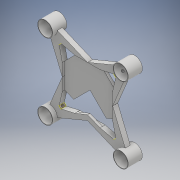
# Autodesk Inventor part: DRONE
Saved by Autodesk Inventor 2018 (Build 220112000, 112)
## iProperties
Created: 2022-03-15
Part Number: DRONE
Material: Genérico
Document SubType Name: Modeling
Designer: ADM
Density: 1 g/cm^3
Appearance: Padrão
Author: ADM
Autodesk Inventor part; units mm, degrees
ref_plane "YZ Plane" through (0, 0, 0) normal (1, 0, 0) x (0, 1, 0)
ref_plane "XZ Plane" through (0, 0, 0) normal (0, 1, 0) x (-1, 0, 0)
ref_plane "XY Plane" through (0, 0, 0) normal (0, 0, 1) x (1, 0, 0)
sketch "Esboço1" plane through (0, 0, 0) normal (0, 1, 0) x (-1, 0, 0)
  line L0 (0, 0) -> (0, -150)
  line L1 (0, 0) -> (150, 0)
  line L2 (150, 0) -> (150, -150)
  line L3 (150, -150) -> (0, -150)
  circle A0 centre (150, -150) radius 15
  circle A1 centre (0, -150) radius 15
  circle A2 centre (0, 0) radius 15
  circle A3 centre (150, 0) radius 15
  line L4 (0, 0) -> (150, -150)
  line L5 (150, 0) -> (0, -150)
  line L6 (75, -75) -> (75, -125)
  line L7 (75, -125) -> (75, -25)
  line L8 (75, -75) -> (125, -75)
  line L9 (75, -25) -> (25, -25)
  line L10 (25, -25) -> (25, -75)
  line L11 (25, -75) -> (25, -125)
  line L12 (25, -125) -> (75, -125)
  line L13 (75, -125) -> (125, -125)
  line L14 (125, -125) -> (125, -75)
  line L15 (125, -75) -> (125, -25)
  line L16 (125, -25) -> (75, -25)
  line L17 (135, -150) -> (75, -125)
  line L18 (125, -75) -> (150, -135)
  line L19 (135, 0) -> (75, -25)
  line L20 (150, -15) -> (125, -75)
  line L21 (15, 0) -> (75, -25)
  line L22 (0, -15) -> (25, -75)
  line L23 (0, -135) -> (25, -75)
  line L24 (15, -150) -> (75, -125)
  line L25 (10.6066, -10.6066) -> (17.6777, -17.6777)
  line L26 (17.6777, -17.6777) -> (50, -25)
  line L27 (17.6777, -17.6777) -> (25, -50)
  line L28 (10.6066, -139.3934) -> (17.6777, -132.3223)
  line L29 (17.6777, -132.3223) -> (25, -100)
  line L30 (17.6777, -132.3223) -> (50, -125)
  line L31 (139.3934, -10.6066) -> (132.3223, -17.6777)
  line L32 (132.3223, -17.6777) -> (100, -25)
  line L33 (132.3223, -17.6777) -> (125, -50)
  line L34 (139.3934, -139.3934) -> (132.3223, -132.3223)
  line L35 (132.3223, -132.3223) -> (125, -100)
  line L36 (132.3223, -132.3223) -> (100, -125)
  dimension "d45" = 150
  dimension "d46" = 150
  dimension "d47" = 150
  dimension "d48" = 30
  dimension "d49" = 30
  dimension "d50" = 30
  dimension "d51" = 30
  dimension "d52" = 50
  dimension "d53" = 100
  dimension "d54" = 50
  dimension "d55" = 100
  dimension "d56" = 50
  dimension "d57" = 50
  dimension "d58" = 50
  dimension "d59" = 50
  dimension "d60" = 10
  dimension "d61" = 10
  dimension "d62" = 10
  dimension "d63" = 10
  constraints: 72 end point, 16 point on line, 12 point on circle, 8 midpoint, 4 centre point, 4 coincident, 2 horizontal, 2 vertical, 1 perpendicular, 10 other
  measures "d45" distance of L0.start L0.end
  measures "d46" distance of L0.start L1.end
  measures "d47" distance of L1.end L2.end
  measures "d48" diameter of A0
  measures "d49" diameter of A1
  measures "d50" diameter of A2
  measures "d51" diameter of A3
  measures "d52" distance of L6.start L6.end
  measures "d53" distance of L6.end L7.end
  measures "d54" distance of L6.start L8.end
  measures "d55" distance of L8.end L10.end
  measures "d56" distance of L7.end L9.end
  measures "d57" distance of L10.end L11.end
  measures "d58" distance of L6.end L13.end
  measures "d59" distance of L8.end L15.end
  measures "d60" distance of L25.start L25.end
  measures "d61" distance of L28.start L28.end
  measures "d62" distance of L31.start L31.end
  measures "d63" distance of L34.start L34.end
extrude "Extrusão1" add sketch "Esboço1" along normal mid plane 28 contours L4 A2 L0 | L0 A2 L1 | L1 A2 L4 | A1 L5 L0 | L0 L3 A1 | A3 L2 L1 | L1 L5 A3 | L5 A1 L3 | L2 A3 L5 | A0 L4 L3 | L3 L2 A0 | L4 A0 L2
extrude "Extrusão2" add sketch "Esboço1" along normal mid plane 10 contours A2 L4 L27 L10 L22 | L21 L9 L26 L4 A2 | L23 L11 L29 L5 A1 | A3 L5 L32 L16 L19 | L5 L30 L12 L24 A1 | A3 L20 L15 L33 L5 | L17 L13 L36 L4 A0 | L18 A0 L4 L35 L14
sketch "Esboço2" plane through (0, -5, 0) normal (0, -1, 0) x (1, 0, 0)
  line L0 (-75, -25) -> (-100, -25) projected
  line L1 (-25.0044, -125) -> (-124.5405, -125)
  line L2 (-132.3223, -132.3223) -> (-125, -100) projected
  line L3 (-17.6777, -132.3223) -> (-25, -100) projected
  line L4 (-125, -50) -> (-125, -75) projected
  line L5 (-125, -50) -> (-74.7992, -75.1004)
  line L6 (-50, -125) -> (-17.6777, -132.3223) projected
  line L7 (-74.7992, -75.1004) -> (-25, -100)
  line L8 (-124.5405, -125) -> (-25.0044, -125)
  line L9 (-74.7725, -125) -> (-25.0044, -125)
  point P0 (0, 0)
  point P1 (-100, -125)
  constraints: 10 end point, 3 collinear, 1 midpoint, 1 parallel
extrude "Extrusão3" add sketch "Esboço1" along normal blind 5 contours L10 L4 L5 L11 | L16 L5 L7 | L7 L4 L9 | L8 L14 L4
extrude "Extrusão4" add sketch "Esboço1" along normal blind 5 contours A3 L20 L15 L33 L5 | L5 L15 L8
sketch "Esboço3" plane through (0, -5, 0) normal (0, -1, 0) x (1, 0, 0)
  line L0 (-100, -125) -> (-75, -125) projected
  line L1 (-75, -125) -> (-75, -115)
  line L2 (-132.3223, -132.3223) -> (-100, -125) projected
  line L3 (-75, -115) -> (-100, -125)
  line L4 (-50, -125) -> (-17.6777, -132.3223) projected
  line L5 (-75, -115) -> (-50, -125)
  point P0 (0, 0)
  dimension "d72" = 10
  constraints: 6 end point, 1 vertical
  measures "d72" distance of L0.end L1.end
extrude "Extrusão5" add sketch "Esboço3" against normal blind 5
sketch "Esboço4" plane through (0, -5, 0) normal (0, -1, 0) x (1, 0, 0)
  line L0 (-75, -125) -> (-75, -115) projected
  line L1 (-50, -125) -> (-17.6777, -132.3223) projected
  line L2 (-75, -115) -> (-50, -125)
  line L3 (-50, -125) -> (-17.6777, -132.3223)
  line L4 (-25, -75) -> (-25, -100) projected
  line L5 (-17.6777, -132.3223) -> (-25, -100)
  line L6 (-25, -125) -> (-124.7945, -125)
  line L7 (-75, -115) -> (-100, -125) projected
  line L8 (-135, -150) -> (-75, -125) projected
  line L9 (-75, -115) -> (-75, -125)
  line L10 (-75, -125) -> (-50, -125)
  line L11 (-75, -125) -> (-50, -125) projected
  line L12 (-50, -125) -> (-75, -125)
  point P0 (0, 0)
  constraints: 14 end point, 1 collinear, 1 horizontal, 1 perpendicular, 1 vertical
extrude "Extrusão6" add sketch "Esboço4" against normal blind 5 contours L0 L2 L6
sketch "Esboço5" plane through (-150, -14, -150) normal (0, -1, 0) x (1, 0, 0)
  circle A0 centre (150, 150) radius 14
  circle A1 centre (-0.0474, 150) radius 14
  circle A2 centre (0, 0) radius 14
  circle A3 centre (150, 0) radius 14
  dimension "d77" = 28
  dimension "d78" = 28
  dimension "d79" = 28
  dimension "d80" = 28
  constraints: 4 centre point, 1 coincident
  measures "d77" diameter of A0
  measures "d78" diameter of A1
  measures "d79" diameter of A2
  measures "d80" diameter of A3
hole "Furo1" at (0, -14, 0) at (-150.0474, -14, 0) at (-150, -14, -150) at (0, -14, -150) direction (0, 1, 0) diameter 28 depth 26 tip angle 118
chamfer "Chanfro1" distance 5 angle 45 4 edges at (-17.6777, 0, -17.6777) (-17.6777, 0, -132.3223) (-132.3223, 0, -132.3223) (-132.3223, 0, -17.6777)
ref_plane "Plano de trabalho1" through (-131.2176, -5, -22.5541) normal (0.7071068, 0, -0.7071068) x (-0.7071068, 0, -0.7071068)
sketch "Esboço6" plane through (-131.2176, -5, -22.5541) normal (0.7071068, 0, -0.7071068) x (-0.7071068, 0, -0.7071068)
  circle A0 centre (-2.6721, 5) radius 2.5
  point P0 (-108.733, 5)
  dimension "d92" = 5
  constraints: 1 centre point
  measures "d92" diameter of A0
hole "Furo2" at (-129.3282, 0, -20.6646) direction (-0.7071068, 0, 0.7071068) diameter 5 depth 20 tip angle 118
ref_plane "Plano de trabalho2" through (-18.7824, -5, -127.4459) normal (-0.7071068, 0, 0.7071068) x (0.7071068, 0, 0.7071068)
sketch "Esboço7" plane through (-18.7824, -5, -127.4459) normal (-0.7071068, 0, 0.7071068) x (0.7071068, 0, 0.7071068)
  circle A0 centre (-2.678, 5) radius 2.5
  point P0 (103.399, 5)
  dimension "d101" = 5
  constraints: 1 centre point
  measures "d101" diameter of A0
hole "Furo3" at (-20.676, 0, -129.3395) direction (0.7071068, 0, -0.7071068) diameter 5 depth 20 tip angle 118
ref_plane "Plano de trabalho3" through (-18.7824, -5, -22.5541) normal (-0.7071068, 0, -0.7071068) x (-0.7071068, 0, 0.7071068)
sketch "Esboço8" plane through (-18.7824, -5, -22.5541) normal (-0.7071068, 0, -0.7071068) x (-0.7071068, 0, 0.7071068)
  circle A0 centre (2.667, 5) radius 2.5
  dimension "d110" = 5
  constraints: 1 centre point, 1 coincident
  measures "d110" diameter of A0
hole "Furo4" at (-20.6682, 0, -20.6682) direction (0.7071068, 0, 0.7071068) diameter 5 depth 20 tip angle 118
ref_plane "Plano de trabalho4" through (-127.4459, -5, -131.2176) normal (0.7071068, 0, 0.7071068) x (0.7071068, 0, -0.7071068)
sketch "Esboço9" plane through (-127.4459, -5, -131.2176) normal (0.7071068, 0, 0.7071068) x (0.7071068, 0, -0.7071068)
  circle A0 centre (-2.667, 5) radius 2.5
  dimension "d119" = 5
  constraints: 1 centre point, 1 coincident
  measures "d119" diameter of A0
hole "Furo5" at (-129.3318, 0, -129.3318) direction (-0.7071068, 0, -0.7071068) diameter 5 depth 20 tip angle 118
chamfer "Chanfro2" distance 25 angle 45 4 edges at (-25, 2.5, -25) (-25, 2.5, -125) (-125, 2.5, -125) (-125, 2.5, -25)
